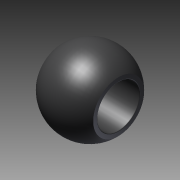
# Autodesk Inventor part: POS 14ECBall
Saved by Autodesk Inventor 2011 SP1 (Build 150282100, 282)
## iProperties
Created: 2017-09-07
Part Number: POS 14ECBall
Catalog Web Link: www.cadenas.de
Description: re_with_m_thread_BA-
Vendor: IKO
Document SubType Name: Modeling
Designer: psAdmin
Manufacturer: IKO
Mass: 4.9354 g
Surface Area: 24.8794 cm^2
Volume: 4.9354 cm^3
Density: 1 g/cm^3
Category: PARTsolutions
Company: IKO
Title: POS 14ECBall
Author: Cadenas PARTsolutions
PSOL_IDENT_0: {$CADENAS_DATA\23d-libs\iko\iko_bearings\pillobals\maintenance_free_type\re_with_m_thread_ba.prj},17
PSOL_IDENT_1: 9 {VTYP=3D},{NB=POS 14ECBall},{LINA=POS 14ECBall},{NN=re_with_m_thread_BA},{DATE=13.10.2016 10:02:13
PSOL_IDENT_2: },{GEOMDATE=02.01.2008 14:02:00},{VERSION=},{LINEID=80},{LINESUBID=-1},{WBVAR=}  {NB=POS 14ECBall},{
PSOL_IDENT_3: LINA=POS 14ECBall},{KT=DUMMY},{IDNR=},{STDRT=14},{ORDER=POS 14EC},{MASS=126.0},{SD=14},{G=M14x2},{ND
PSOL_IDENT_4: M=14},{P1=2.00},{SD2=34},{C1=13.50},{B=19},{SD1=16.9},{SL2=77},{SH=60},{SL1=36},{SR1=0.2},{SDK=25.40
PSOL_IDENT_5: 0},{D4=28.1059},{C2=7.5001},{C3=7.5},{AA=0.0000},{BB=0},{R2=4.0},{R3=26.0},{R4=16.7669},{C=60},{LL6=
PSOL_IDENT_6: 38.25},{LL7=41.5},{LL8=2.4249},{LL9=0.0000},{LL10=0.0000},{LL11=75.6000},{CD=33600},{CS=17200},{SL10=
PSOL_IDENT_7: 0.0000},{G1=14},{GG1=11.835},{PP=2.00},{BL=2},{SC=1},{DBL=25.40}
NN: re_with_m_thread_BA
NB: POS 14ECBall
NBSYN: $ORDER.Ball
LINA: POS 14ECBall
STDRT: 14
ORDER: POS 14EC
MASS: 126.0
SD: 14
G: M14x2
NDM: 14
P1: 2.00
SD2: 34
C1: 13.50
B: 19
SD1: 16.9
SL2: 77
SH: 60
SL1: 36
SR1: 0.2
SDK: 25.400
D4: 28.1059
C2: 7.5001
C3: 7.5
AA: 0.0000
BB: 0
R2: 4.0
R3: 26.0
R4: 16.7669
C: 60
LL6: 38.25
LL7: 41.5
LL8: 2.4249
LL9: 0.0000
LL10: 0.0000
LL11: 75.6000
CD: 33600
CS: 17200
SL10: 0.0000
G1: 14
GG1: 11.835
PP: 2.00
BL: 2
SC: 1
DBL: 25.40
SUPPLIER: IKO
ARTICLENO: POS 14ECBall
BOMINFO: POS 14ECBall
CREATOR: CADENAS GmbH
Autodesk Inventor part; units mm, degrees
ref_plane "YZ Plane" through (0, 0, 0) normal (1, 0, 0) x (0, 1, 0)
ref_plane "XZ Plane" through (0, 0, 0) normal (0, 1, 0) x (-1, 0, 0)
ref_plane "XY Plane" through (0, 0, 0) normal (0, 0, 1) x (1, 0, 0)
sketch "Sketch_1" plane through (0, 0, 0) normal (0, 0, 1) x (1, 0, 0)
  line L0 (19, 0) -> (0, 0)
  arc A0 (0, 7.2) -> (0.2, 7) centre (0.2, 7.2) ccw
  line L1 (0.2, 7) -> (18.8, 7)
  arc A1 (18.8, 7) -> (19, 7.2) centre (18.8, 7.2) ccw
  line L2 (19, 7.2) -> (19, 8.45)
  arc A2 (19, 8.45) -> (0, 8.45) centre (9.5, 0.0215) ccw
  line L3 (0, 8.45) -> (0, 7.2)
  constraints: 8 end point, 6 point on circle, 3 centre point
revolve "Revolution1" add sketch "Sketch_1" angle 360 about axis through (19, 0, 0) along (1, 0, 0)
ref_plane "IP_1_BA_XY" through (9.5, 0, 0) normal (1, 0, 0) x (0, 0, -1)
ref_plane "IP_1_BA_YZ" through (9.5, 0, 0) normal (0, 0, -1) x (0, 1, 0)
ref_plane "IP_1_BA_ZX" through (9.5, 0, 0) normal (0, 1, 0) x (1, 0, 0)
body "Solid1"
